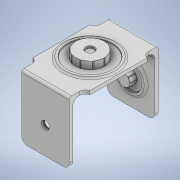
# Autodesk Inventor part: мотор_плеча_2v2
Saved by Autodesk Inventor 2022 (Build 260153000, 153)
## iProperties
Created: 2022-12-04
Part Number: мотор_плеча_2v2
Material: Типовые
Document SubType Name: Modeling
Designer: Папа
Density: 1 g/cm^3
Appearance: По умолчанию
Author: Папа
Autodesk Inventor part; units mm, degrees
ref_plane "YZ Plane" through (0, 0, 0) normal (1, 0, 0) x (0, 1, 0)
ref_plane "XZ Plane" through (0, 0, 0) normal (0, 1, 0) x (-1, 0, 0)
sketch "Эскиз1" plane through (0, 0, 0) normal (0, 1, 0) x (-1, 0, 0)
  line L0 (-20, -37.5) -> (20, -37.5)
  line L1 (20, -37.5) -> (20, 37.5)
  line L2 (20, 37.5) -> (-20, 37.5)
  line L3 (-20, 37.5) -> (-20, -37.5)
  line L4 (-20, -37.5) -> (20, 37.5) construction
  line L5 (20, -37.5) -> (-20, 37.5) construction
  point P0 (0, 0)
  dimension "d0" = 40
  dimension "d1" = 75
  constraints: 12 end point, 2 midpoint, 2 parallel, 1 horizontal, 1 perpendicular
  measures "d0" distance between parallel lines of L3 L1
  measures "d1" distance of L0.end L1.end
extrude "Выдавливание1" add sketch "Эскиз1" along normal blind 3
sketch "Эскиз2" plane through (0, 3, 0) normal (0, 1, 0) x (1, 0, 0)
  circle A0 centre (0, 0) radius 18.9
  circle A1 centre (0, 0) radius 20.9
  dimension "d4" = 37.8
  dimension "d5" = 2
  constraints: 2 centre point, 2 coincident
  measures "d4" diameter of A0
  measures "d5" radial gap between concentric circles of A0 A1
extrude "Выдавливание2" add sketch "Эскиз2" along normal blind 1
sketch "Эскиз3" plane through (0, 3, 0) normal (0, 1, 0) x (1, 0, 0)
  circle A0 centre (0, 0) radius 12.1
  dimension "d9" = 24.2
  constraints: 1 centre point, 1 coincident
  measures "d9" diameter of A0
extrude "Выдавливание3" add sketch "Эскиз3" along normal blind 6
sketch "Эскиз5" plane through (0, 0, 0) normal (0, -1, 0) x (1, 0, 0)
  line L0 (24, 24) -> (24, -24)
  line L1 (24, -24) -> (-24, -24)
  line L2 (-24, -24) -> (-24, 24)
  line L3 (-24, 24) -> (24, 24)
  circle A0 centre (0, 0) radius 12.5
  dimension "d16" = 48
  dimension "d17" = 25
  constraints: 8 end point, 2 coincident, 1 centre point, 1 horizontal, 9 other
  measures "d16" distance of L2.end L0.start
  measures "d17" diameter of A0
extrude "Выдавливание5" add sketch "Эскиз5" against normal blind 3
fillet "Сопряжение1" radius 2 1 edges at (-20.9, 3, 0)
fillet "Сопряжение3" radius 5 4 edges at (20, 1.5, -24) (20, 1.5, 24) (-20, 1.5, 24) (-20, 1.5, -24)
ref_plane "РабПлоскость1" through (20, 0, 0) normal (0, 0, -1) x (-1, 0, 0)
sketch "Эскиз6" plane through (-20, 0, 37.5) normal (0, 0, 1) x (1, 0, 0)
  line L0 (40, 3) -> (44, 3) projected
  line L1 (40, 3) -> (0, 3)
  line L2 (0, 3) -> (0, -50)
  line L3 (0, -50) -> (40, -50)
  line L4 (40, -50) -> (40, 3)
  line L5 (0, 0) -> (40, 0) projected
  point P0 (20, 0)
  dimension "d25" = 50
  constraints: 8 end point, 2 parallel, 1 horizontal, 1 perpendicular, 1 point on line
  measures "d25" distance between parallel lines of L5 L3
extrude "Выдавливание6" add sketch "Эскиз6" against normal blind 3 contours L4 L3 L2 L5
fillet "Сопряжение4" radius 5 1 edges at (0, 0, 34.5)
fillet "Сопряжение5" radius 5 2 edges at (-20, -50, 36) (20, -50, 36)
mirror "Зеркальное отражение2" about plane through (20, 0, 0) normal (0, 0, -1) of "Выдавливание6", "Сопряжение5", "Сопряжение4"
sketch "Эскиз7" plane through (-20, 0, 34.5) normal (0, 0, -1) x (-1, 0, 0)
  line L0 (-40, -45) -> (-40, 3) projected
  line L1 (0, -45) -> (0, 3) projected
  line L2 (0, -5) -> (-40, -5)
  line L3 (-40, -5) -> (-40, -50)
  line L4 (-40, -50) -> (0, -50)
  line L5 (0, -50) -> (0, -5)
  line L6 (-35, -50) -> (-5, -50) projected
  arc A0 (-40, -45) -> (-35, -50) centre (-35, -45) ccw projected
  line L7 (-35, -50) -> (-5, -50) projected
  arc A1 (-5, -50) -> (0, -45) centre (-5, -45) ccw projected
  line L8 (0, -45) -> (0, -5) projected
  line L9 (-40, -5) -> (0, -5) projected
  line L10 (-40, -5) -> (-40, -45) projected
  line L11 (0, -50) -> (-40, -5) construction
  circle A2 centre (-20, -27.5) radius 3.5
  point P0 (-20, 0)
  dimension "d31" = 40
  dimension "d33" = 7
  constraints: 10 end point, 2 collinear, 2 parallel, 1 centre point, 1 horizontal, 1 midpoint, 1 perpendicular, 1 point on line
  measures "d31" distance of L3.end L4.end
  measures "d33" diameter of A2
extrude "Выдавливание7" cut sketch "Эскиз7" against normal blind 3 contours A2
sketch "Эскиз8" plane through (-20, -5, -34.5) normal (0, 0, 1) x (1, 0, 0)
  line L0 (0, 0) -> (40, 0) projected
  line L1 (0, 0) -> (40, 0)
  line L2 (40, 0) -> (40, -45)
  line L3 (40, -45) -> (0, -45)
  line L4 (0, -45) -> (0, 0)
  line L5 (40, 0) -> (0, -45) construction
  line L6 (35, -45) -> (5, -45) projected
  line L7 (40, 0) -> (40, -40) projected
  circle A0 centre (20, -22.5) radius 10.5
  circle A1 centre (20, -22.5) radius 12.5
  point P0 (20, 5)
  dimension "d36" = 21
  dimension "d37" = 2
  constraints: 10 end point, 2 centre point, 2 collinear, 2 parallel, 1 coincident, 1 horizontal, 1 midpoint, 1 perpendicular
  measures "d36" diameter of A0
  measures "d37" radial gap between concentric circles of A1 A0
extrude "Выдавливание8" add sketch "Эскиз8" along normal blind 1.4 contours A1
sketch "Эскиз9" plane through (0, -27.5, -34.5) normal (0, 0, 1) x (1, 0, 0)
  circle A0 centre (0, 0) radius 10.5 projected
  circle A1 centre (0, 0) radius 5
  point P0 (0, 27.5)
  dimension "d40" = 10
  constraints: 1 centre point, 1 coincident
  measures "d40" diameter of A1
extrude "Выдавливание9" add sketch "Эскиз9" along normal blind 6 contours A1
fillet "Сопряжение6" radius 2 1 edges at (-12.5, -27.5, -34.5)
sketch "Эскиз10" plane through (0, -27.5, -28.5) normal (0, 0, 1) x (1, 0, 0)
  circle A0 centre (0, 0) radius 5 projected
  circle A1 centre (-5, 0) radius 0.25
  point P0 (0, 27.5)
  point P1 (-4.9938, -0.2499)
  point P2 (-4.9938, 0.2499)
  dimension "d44" = 0.5
  constraints: 1 centre point, 2 other
  measures "d44" diameter of A1
extrude "Выдавливание10" add sketch "Эскиз10" against normal up to surface (6 mm away) contours A0 A1 picked at (-5.0822, 0.0102)
fillet "Сопряжение7" radius 0.4 2 edges at (-4.9937, -27.2501, -31.5) (-4.9937, -27.7499, -31.5)
pattern_circular "Круговой массив1" count 8 over 360 about axis through (0, -27.5, -34.5) along (0, 0, 1) of "Сопряжение7", "Выдавливание10"
fillet "Сопряжение8" radius 0.2 66 edges at (-3.789, -30.8221, -28.5) (-3.7123, -31.2123, -28.5) (-3.3221, -31.289, -28.5) (-1.9134, -32.1194, -28.5) (-0.3301, -32.5283, -28.5) (0, -32.75, -28.5) (0.3301, -32.5283, -28.5) (1.9134, -32.1194, -28.5) (3.3221, -31.289, -28.5) (3.7123, -31.2123, -28.5) (3.789, -30.8221, -28.5) (4.6194, -29.4134, -28.5) (5.0283, -27.8301, -28.5) (5.25, -27.5, -28.5) (5.0283, -27.1699, -28.5) (4.6194, -25.5866, -28.5) (3.789, -24.1779, -28.5) (3.7123, -23.7877, -28.5) (3.3221, -23.711, -28.5) (1.9134, -22.8806, -28.5) (0.3301, -22.4717, -28.5) (0, -22.25, -28.5) (-0.3301, -22.4717, -28.5) (-1.9134, -22.8806, -28.5) (-3.3221, -23.711, -28.5) (-3.7123, -23.7877, -28.5) (-3.789, -24.1779, -28.5) (-4.6194, -25.5866, -28.5) (-5.0283, -27.1699, -28.5) (-5.25, -27.5, -28.5) (-5.0283, -27.8301, -28.5) (-4.6194, -29.4134, -28.5) (-5.0283, -27.8301, -34.5) (-5.25, -27.5, -34.5) (-5.0283, -27.1699, -34.5) (-4.6194, -25.5866, -34.5) (-3.789, -24.1779, -34.5) (-3.7123, -23.7877, -34.5) (-3.3221, -23.711, -34.5) (-1.9134, -22.8806, -34.5) (-0.3301, -22.4717, -34.5) (0, -22.25, -34.5) (0.3301, -22.4717, -34.5) (1.9134, -22.8806, -34.5) (3.3221, -23.711, -34.5) (3.7123, -23.7877, -34.5) (3.789, -24.1779, -34.5) (4.6194, -25.5866, -34.5) (5.0283, -27.1699, -34.5) (5.25, -27.5, -34.5) (5.0283, -27.8301, -34.5) (4.6194, -29.4134, -34.5) (3.789, -30.8221, -34.5) (3.7123, -31.2123, -34.5) (3.3221, -31.289, -34.5) (1.9134, -32.1194, -34.5) (0.3301, -32.5283, -34.5) (0, -32.75, -34.5) (-0.3301, -32.5283, -34.5) (-1.9134, -32.1194, -34.5) (-3.3221, -31.289, -34.5) (-3.7123, -31.2123, -34.5) (-3.789, -30.8221, -34.5) (-4.6194, -29.4134, -34.5) (-10.5, -27.5, -34.5) (-10.5, -27.5, -33.1)
sketch "Эскиз11" plane through (0, 9, 0) normal (0, 1, 0) x (1, 0, 0)
  circle A0 centre (0, 0) radius 12.1 projected
  circle A1 centre (0, 0) radius 12.1 projected
  circle A2 centre (-12.1, 0) radius 0.25
  dimension "d52" = 0.5
  constraints: 1 centre point, 1 horizontal alignment, 1 other
  measures "d52" diameter of A2
extrude "Выдавливание11" add sketch "Эскиз11" against normal up to surface (6 mm away) contours A2 A0 | A0 A2 picked at (-12.0165, 0) picked at (-12.1825, 0.0101)
fillet "Сопряжение9" radius 0.7 2 edges at (-12.0974, 6, -0.25) (-12.0974, 6, 0.25)
pattern_circular "Круговой массив2" count 10 over 360 about axis through (0, 3, 0) along (0, 1, 0) of "Выдавливание11", "Сопряжение9"
fillet "Сопряжение10" radius 0.2 81 edges at (-12.141, 9, -0.3813) (-12.35, 9, 0) (-12.141, 9, 0.3813) (-11.5078, 9, 3.7391) (-10.0464, 9, 6.8278) (-9.9914, 9, 7.2591) (-9.5982, 9, 7.4448) (-7.1122, 9, 9.7891) (-4.1144, 9, 11.429) (-3.8164, 9, 11.7455) (-3.3892, 9, 11.6646) (0, 9, 12.1) (3.3892, 9, 11.6646) (3.8164, 9, 11.7455) (4.1144, 9, 11.429) (7.1122, 9, 9.7891) (9.5982, 9, 7.4448) (9.9914, 9, 7.2591) (10.0464, 9, 6.8278) (11.5078, 9, 3.7391) (12.141, 9, 0.3813) (12.35, 9, 0) (12.141, 9, -0.3813) (11.5078, 9, -3.7391) (10.0464, 9, -6.8278) (9.9914, 9, -7.2591) (9.5982, 9, -7.4448) (7.1122, 9, -9.7891) (4.1144, 9, -11.429) (3.8164, 9, -11.7455) (3.3892, 9, -11.6646) (0, 9, -12.1) (-3.3892, 9, -11.6646) (-3.8164, 9, -11.7455) (-4.1144, 9, -11.429) (-7.1122, 9, -9.7891) (-9.5982, 9, -7.4448) (-9.9914, 9, -7.2591) (-10.0464, 9, -6.8278) (-11.5078, 9, -3.7391) (-10.0464, 3, -6.8278) (-9.9914, 3, -7.2591) (-9.5982, 3, -7.4448) (-7.1122, 3, -9.7891) (-4.1144, 3, -11.429) (-3.8164, 3, -11.7455) (-3.3892, 3, -11.6646) (0, 3, -12.1) (3.3892, 3, -11.6646) (3.8164, 3, -11.7455) (4.1144, 3, -11.429) (7.1122, 3, -9.7891) (9.5982, 3, -7.4448) (9.9914, 3, -7.2591) (10.0464, 3, -6.8278) (11.5078, 3, -3.7391) (12.141, 3, -0.3813) (12.35, 3, 0) (12.141, 3, 0.3813) (11.5078, 3, 3.7391) (10.0464, 3, 6.8278) (9.9914, 3, 7.2591) (9.5982, 3, 7.4448) (7.1122, 3, 9.7891) (4.1144, 3, 11.429) (3.8164, 3, 11.7455) (3.3892, 3, 11.6646) (0, 3, 12.1) (-3.3892, 3, 11.6646) (-3.8164, 3, 11.7455) (-4.1144, 3, 11.429) (-7.1122, 3, 9.7891) (-9.5982, 3, 7.4448) (-9.9914, 3, 7.2591) (-10.0464, 3, 6.8278) (-11.5078, 3, 3.7391) (-12.141, 3, 0.3813) (-12.35, 3, 0) (-12.141, 3, -0.3813) (-11.5078, 3, -3.7391) (-18.9, 4, 0)
fillet "Сопряжение11" radius 2 2 edges at (0, 3, -37.5) (0, 3, 37.5)
sketch "Эскиз15" plane through (0, 9, 0) normal (0, 1, 0) x (1, 0, 0)
  circle A0 centre (0, 0) radius 3.5
  dimension "d64" = 7
  constraints: 1 centre point, 1 coincident
  measures "d64" diameter of A0
extrude "Выдавливание12" cut sketch "Эскиз15" against normal blind 1.5
fillet "Сопряжение12" radius 0.3 2 edges at (-3.5, 9, 0) (-3.5, 7.5, 0)
